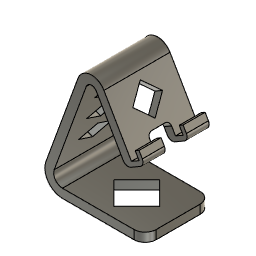
Handyhalterung v6 (Autodesk Fusion 360 design; units mm, degrees)
Autodesk Fusion 360 part; units mm, degrees
sketch "Skizze1" plane through (0, 0, 0) normal (0, 1, 0) x (1, 0, 0)
  line L0 (0, 0) -> (-75.0363, 0)
  line L1 (-90.0714, -21.4723) -> (-60.8666, -101.7116)
  line L2 (0, 0) -> (0, -8)
  line L3 (0, -8) -> (-75.0363, -8)
  line L4 (-82.5538, -18.7362) -> (-53.3491, -98.9755)
  line L5 (-44.3205, -99.7654) -> (-17.3205, -53)
  line L6 (-17.3205, -53) -> (0, -63)
  line L7 (0, -63) -> (-5.5, -72.5263)
  line L8 (-5.5, -72.5263) -> (-8.9641, -70.5263)
  line L9 (-8.9641, -70.5263) -> (-5.4641, -64.4641)
  line L10 (-5.4641, -64.4641) -> (-12.3923, -60.4641)
  line L11 (-12.3923, -60.4641) -> (-37.3923, -103.7654)
  arc A0 (-53.3491, -98.9755) -> (-44.3205, -99.7654) centre (-48.6506, -97.2654) ccw
  arc A1 (-60.8666, -101.7116) -> (-37.3923, -103.7654) centre (-48.6506, -97.2654) ccw
  arc A2 (-75.0363, 0) -> (-90.0714, -21.4723) centre (-75.0363, -16) ccw
  arc A3 (-75.0363, -8) -> (-82.5538, -18.7362) centre (-75.0363, -16) ccw
  dimension "d3" = 8
  dimension "d4" = 8
  dimension "d5" = 8
  dimension "d7" = 30
  dimension "d8" = 4
  dimension "d10" = 4
  dimension "d11" = 8
  dimension "d12" = 7
  dimension "d19" = 70
  dimension "d20" = 50
  dimension "d21" = 5
  dimension "d23" = 8
  dimension "d24" = 45
  constraint coincident L0.start L2.start
  constraint horizontal L0
  constraint perpendicular L0 L2
  constraint perpendicular L2 L3
  constraint perpendicular L6 L7
  constraint perpendicular L7 L8
  constraint perpendicular L6 L9
  constraint perpendicular L9 L10
  constraint parallel L5 L11
  constraint parallel L1 L4
  constraint tangent L5 A0
  constraint tangent L11 A1
  constraint tangent L1 A1
  constraint tangent L4 A0
  constraint concentric A0 A1
  constraint parallel L9 L11
  constraint tangent L0 A2
  constraint tangent L1 A2
  constraint tangent L3 A3
  constraint tangent L4 A3
  constraint coincident L2 L6.end
  constraint concentric A2 A3
  measures "d3" distance of L0.start L2.end
  measures "d4" distance of L1 L4
  measures "d5" distance of L5 L11
  measures "d7" angle of L2 L11
  measures "d8" distance of L6 L10
  measures "d10" distance of L7 L9
  measures "d11" distance of L9 L11
  measures "d12" distance of L8.end L9.end
  measures "d19" angle of L3 L4
  measures "d20" distance of L10.end L11.end
  measures "d21" radius of A0
  measures "d23" radius of A3
  measures "d24" distance of L3 L5.end
extrude "Extrusion1" add sketch "Skizze1" along normal mid plane 60
fillet "Abrundung1" radius 10 2 edges at (0, 30, 4) (0, -30, 4)
fillet "Abrundung2" radius 5 2 edges at (-17.3205, 0, 53) (0, 0, 63)
sketch "Skizze2" plane through (-86.4361, 0, 31.4602) normal (-0.939693, 0, 0.34202) x (0, -1, 0)
  line L0 (30, 74.7601) -> (-30, 74.7601)
  line L1 (-30, 74.7601) -> (-30, -10.6288)
  line L2 (-30, -10.6288) -> (30, -10.6288)
  line L3 (30, -10.6288) -> (30, 74.7601)
  line L4 (37, 74.7601) -> (69, 74.7601) construction
  line L5 (40.6572, -10.6288) -> (65.6572, -10.6288) construction
  line L6 (0, 60.3905) -> (-15, 53.4128)
  line L7 (-15, 53.4128) -> (0, 46.4352)
  line L8 (0, 46.4352) -> (15, 53.4128)
  line L9 (15, 53.4128) -> (0, 60.3905)
  line L10 (0, 96) -> (0, -24.4616) construction
  line L11 (-15, 32.0656) -> (0, 39.0433)
  line L12 (15, 32.0656) -> (0, 25.0879)
  line L13 (0, 25.0879) -> (-15, 32.0656)
  line L14 (0, 39.0433) -> (15, 32.0656)
  line L15 (-15, 10.7184) -> (0, 17.6961)
  line L16 (15, 10.7184) -> (0, 3.7407)
  line L17 (0, 17.6961) -> (15, 10.7184)
  line L18 (0, 3.7407) -> (-15, 10.7184)
  line L19 (54.5845, 53.4128) -> (42.5845, 53.4128) construction
  line L20 (44.9665, 10.7184) -> (55.9665, 10.7184) construction
  line L21 (44.2293, 32.0656) -> (77.6613, 32.0656) construction
  line L22 (-30, 117.5218) -> (-30, 95) construction
  line L23 (30, 116.8852) -> (30, 115.0039)
  line L24 (30, 115.0039) -> (30, 98.1735) construction
  line L25 (-15, 115.7395) -> (-15, 115.0001)
  line L26 (-15, 115.0001) -> (-15, 100.3356) construction
  line L27 (15, 114.7211) -> (15, 98.5535) construction
  dimension "d61" = 90.7098
  dimension "d62" = 13.9554
  dimension "d63" = 13.9554
  dimension "d64" = 13.9554
  constraint perpendicular L3 L4
  constraint perpendicular L3 L5
  constraint collinear L0 L4
  constraint collinear L2 L5
  constraint coincident L6.start L10
  constraint coincident L7.end L10
  constraint coincident L10 L15.end
  constraint coincident L10 L11.end
  constraint coincident L10 L12.end
  constraint coincident L10 L16.end
  constraint coincident L11.start L13.end
  constraint perpendicular L3 L19
  constraint symmetric L6.start L7.end L19
  constraint coincident L8.end L19
  constraint coincident L6.end L19
  constraint perpendicular L3 L20
  constraint coincident L11.start L21
  constraint coincident L12.start L21
  constraint coincident L15.start L20
  constraint coincident L16.start L20
  constraint symmetric L16.end L15.end L20
  constraint symmetric L11.end L12.end L21
  constraint vertical L22
  constraint vertical L23
  constraint parallel L23 L24
  constraint collinear L3 L24
  constraint collinear L1 L22
  constraint parallel L22 L25
  constraint parallel L22 L26
  constraint vertical L27
  constraint coincident L8.end L27
  constraint coincident L12.start L27
  constraint coincident L16.start L27
  constraint coincident L6.end L26
  constraint coincident L11.start L26
  constraint coincident L15.start L26
  measures "d62" distance of L6.start L7.end
  measures "d63" distance of L11.end L12.end
  measures "d64" distance of L16.end L15.end
sketch "Skizze3" plane through (0, 0, 0) normal (0, 0, -1) x (1, 0, 0)
  arc A0 (0, 20) -> (-10, 30) centre (-10, 20) ccw
  line L0 (-10, 30) -> (-75.0363, 30)
  line L1 (-75.0363, 30) -> (-75.0363, -30)
  line L2 (-75.0363, -30) -> (-10, -30)
  arc A1 (-10, -30) -> (0, -20) centre (-10, -20) ccw
  line L3 (0, -20) -> (0, 20)
  line L4 (-37.5181, 20.7692) -> (-16.7489, 0)
  line L5 (-16.7489, 0) -> (-37.5181, -20.7692)
  line L6 (-37.5181, -20.7692) -> (-58.2874, 0)
  line L7 (-58.2874, 0) -> (-37.5181, 20.7692)
  line L8 (14.0727, 0) -> (33.0727, 0) construction
  line L9 (16, 30) -> (33.0294, 30) construction
  line L10 (13, -30) -> (35, -30) construction
  line L11 (-37.5181, 48.9997) -> (-37.5181, 36.9997) construction
  line L12 (-75.0363, 50.8097) -> (-75.0363, 32.3583) construction
  line L13 (0, 50.8507) -> (0, 32.3183) construction
  dimension "d65" = 41.5385
  dimension "d66" = 60
  constraint perpendicular L4 L5
  constraint parallel L4 L6
  constraint parallel L5 L7
  constraint horizontal L8
  constraint perpendicular L3 L10
  constraint collinear L0 L9
  constraint collinear L2 L10
  constraint coincident L4.end L8
  constraint coincident L6.end L8
  constraint coincident L4.start L11
  constraint coincident L5.end L11
  constraint collinear L3 L13
  constraint collinear L1 L12
  measures "d65" distance of L4.start L5.end
  measures "d66" distance of L9 L10
sketch "Skizze4" plane through (0, 0, 0) normal (0, 1, 0) x (1, 0, 0)
  line L0 (-7.5, -75.9904) -> (-24.8205, -65.9904)
  line L1 (-24.8205, -65.9904) -> (-17.3205, -53)
  line L2 (-17.3205, -53) -> (0, -63)
  line L3 (0, -63) -> (-7.5, -75.9904)
  line L4 (-4.3301, -60.5) -> (-12.9904, -55.5)
  line L5 (-5.5, -72.5263) -> (-2.5, -67.3301)
  line L6 (-19.8205, -57.3301) -> (-44.3205, -99.7654)
  dimension "d68" = 15
  constraint perpendicular L0 L1
  constraint perpendicular L1 L2
  constraint perpendicular L2 L3
  constraint coincident L0.start L3.end
  constraint parallel L0 L4
  constraint collinear L3 L5
  constraint collinear L1 L6
  constraint collinear L2 L4
  measures "d68" distance of L2.end L0.start
extrude "Extrusion2" cut sketch "Skizze4" along normal mid plane 20
fillet "Abrundung3" radius 4 2 edges at (-21.3564, 10, 67.9904) (-21.3564, -10, 67.9904)
sketch "Skizze5" plane through (16.8875, 0, 9.75) normal (0.866025, 0, 0.5) x (0, 1, 0)
  line L0 (10, 65.5596) -> (10, 58.5596)
  line L1 (10, 58.5596) -> (30, 58.5596)
  line L2 (30, 58.5596) -> (30, 108.5596)
  line L3 (30, 108.5596) -> (-30, 108.5596)
  line L4 (-30, 108.5596) -> (-30, 58.5596)
  line L5 (-30, 58.5596) -> (-10, 58.5596)
  line L6 (-10, 58.5596) -> (-10, 65.5596)
  arc A0 (-6, 69.5596) -> (-10, 65.5596) centre (-6, 65.5596) ccw
  line L7 (-6, 69.5596) -> (6, 69.5596)
  arc A1 (10, 65.5596) -> (6, 69.5596) centre (6, 65.5596) ccw
  line L8 (13.5, 89.0596) -> (0, 102.5596)
  line L9 (0, 102.5596) -> (-13.5, 89.0596)
  line L10 (-13.5, 89.0596) -> (0, 75.5596)
  line L11 (0, 75.5596) -> (13.5, 89.0596)
  line L12 (13.5, 89.0596) -> (-13.5, 89.0596) construction
  line L13 (0, 102.5596) -> (0, 75.5596) construction
  line L14 (0, 132.171) -> (0, 54.7397)
  line L15 (57, 89.0596) -> (43, 89.0596) construction
  line L16 (42, 108.5596) -> (57, 108.5596) construction
  line L17 (43, 69.5596) -> (60, 69.5596) construction
  point P0 (0, 89.0596)
  dimension "d73" = 39
  dimension "d74" = 27
  constraint perpendicular L8 L9
  constraint parallel L8 L10
  constraint parallel L9 L11
  constraint coincident L12 P0
  constraint coincident L13 P0
  constraint coincident P0 L14
  constraint coincident L8.end L14
  constraint horizontal L15
  constraint horizontal L16
  constraint horizontal L17
  constraint collinear L7 L17
  constraint collinear L3 L16
  constraint collinear L12 L15
  measures "d73" distance of L16 L17
  measures "d74" distance of L8.end L10.end
extrude "Extrusion3" cut sketch "Skizze5" against normal up to surface (8 mm away) contours L8 L11 L14 | L9 L10 L14
extrude "Extrusion4" cut sketch "Skizze3" against normal up to surface (8 mm away) contours L4 L5 L6 L7
extrude "Extrusion5" cut sketch "Skizze2" against normal up to surface (8 mm away) contours L6 L7 L8 L9 | L11 L12 L13 L14 | L15 L16 L17 L18
equation "angle = 30 deg"
equation "d4 = d3"
equation "d5 = d3"
equation "d7 = angle"
equation "d8 = d3 / 2"
equation "thickness = 8 mm"
equation "d10 = d8"
equation "d11 = thickness"
equation "d12 = bracket_depth"
equation "bracket_depth = 7 mm"
equation "length = 150 mm"
equation "width = 60 mm"
equation "cable_width = 20 mm"
equation "d20 = length / 3"
equation "d24 = platform_height"
equation "platform_height = 45 mm"
equation "d26 = width / 2"
equation "d50 = 45.35489 mm / 3"
equation "d53 = 90.709781 mm / 13"
equation "d54 = d53"
equation "d56 = 90.709781 mm * 3 / 14"
equation "d62 = 90.709781 mm * 2 / 13"
equation "d63 = d62"
equation "d64 = d62"
equation "d65 = 60.00 mm * 9 / 13"
equation "d69 = cable_width / 2"
equation "d74 = 39.00 mm * 9 / 13"
